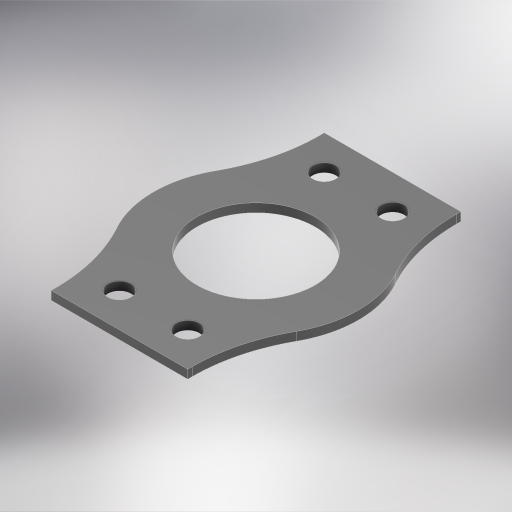
# Autodesk Inventor part: ball bearing holder
Saved by Autodesk Inventor 2023 (Build 270158000, 158)
## iProperties
Created: 2022-10-31
Part Number: ball bearing holder
Material: Acetal Resin, Black
Document SubType Name: Modeling
Designer: aaron
Density: 1.425 g/cm^3
Appearance: Smooth - Black
Author: aaron
Autodesk Inventor part; units mm, degrees
ref_plane "YZ Plane" through (0, 0, 0) normal (1, 0, 0) x (0, 1, 0)
ref_plane "XZ Plane" through (0, 0, 0) normal (0, 1, 0) x (-1, 0, 0)
ref_plane "XY Plane" through (0, 0, 0) normal (0, 0, 1) x (1, 0, 0)
sketch "Sketch1" plane through (0, 0, 0) normal (0, 1, 0) x (-1, 0, 0)
  circle A0 centre (0, 0) radius 10.9855
  line L0 (12.7, -25.4) -> (-12.7, -25.4)
  line L1 (-12.7, -25.4) -> (-12.7, 25.4)
  line L2 (-12.7, 25.4) -> (12.7, 25.4)
  line L3 (12.7, 25.4) -> (12.7, -25.4)
  line L4 (12.7, -25.4) -> (-12.7, 25.4) construction
  line L5 (-12.7, -25.4) -> (12.7, 25.4) construction
  circle A1 centre (0, 0) radius 19.05
  circle A2 centre (-6.35, -19.05) radius 2.159
  circle A3 centre (6.35, -19.05) radius 2.159
  circle A4 centre (-6.35, 19.05) radius 2.159
  circle A5 centre (6.35, 19.05) radius 2.159
  point P0 (-12.7, -14.199)
  point P1 (12.7, -14.199)
  point P2 (12.7, 14.199)
  point P3 (-12.7, 14.199)
  dimension "d0" = 21.971
  dimension "d1" = 25.4
  dimension "d2" = 50.8
  dimension "d3" = 38.1
  dimension "d4" = 4.318
  dimension "d5" = 6.35
  dimension "d6" = 6.35
  dimension "d9" = 12.7
  dimension "d12" = 38.1
  constraints: 12 end point, 6 centre point, 2 coincident, 2 horizontal, 2 midpoint, 2 parallel, 1 perpendicular, 1 vertical, 6 other
  measures "d0" diameter of A0
  measures "d1" distance of L1.end L2.end
  measures "d2" distance of L0.end L1.end
  measures "d3" diameter of A1
  measures "d4" diameter of A2
  measures "d5" distance from line of L0 A2.centre
  measures "d6" distance from line of L1 A2.centre
  measures "d9" distance of A2.centre A3.centre
  measures "d12" distance of A2.centre A4.centre
extrude "Extrusion1" add sketch "Sketch1" along normal blind 1.5875 contours L0 L1 A1 A2 A3 L3 | A1 A3 A2 L1 A4 A5 L3 | L3 A1 | A1 L1 | A1 A5 A4 L1 L2 L3
fillet "Fillet1" radius 31.75 4 edges at (12.7, 0.7937, 14.199) (12.7, 0.7937, -14.199) (-12.7, 0.7937, -14.199) (-12.7, 0.7937, 14.199)
body "Solid1"
